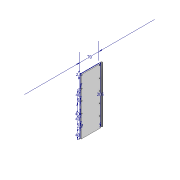
# Autodesk Inventor part: SidePanel
Saved by Autodesk Inventor 2020.3 (Build 243373010, 373A)
## iProperties
Created: 2020-12-03
Part Number: SidePanel
Material: Generic
Document SubType Name: Modeling
Designer: Yusuf
Mass: 79.5373 g
Surface Area: 369.992 cm^2
Volume: 79.5373 cm^3
Density: 1 g/cm^3
Appearance: Default
Author: Yusuf
Autodesk Inventor part; units mm, degrees
ref_plane "YZ Plane" through (0, 0, 0) normal (1, 0, 0) x (0, 1, 0)
ref_plane "XZ Plane" through (0, 0, 0) normal (0, 1, 0) x (-1, 0, 0)
ref_plane "XY Plane" through (0, 0, 0) normal (0, 0, 1) x (1, 0, 0)
sketch "Sketch1" plane through (0, 0, 0) normal (1, 0, 0) x (0, 1, 0)
  line L0 (0, 0) -> (205, 0)
  line L1 (205, 0) -> (205, -70)
  line L2 (205, -70) -> (0, -70)
  line L3 (0, -70) -> (0, 0)
  circle A0 centre (40, -2.5) radius 1
  circle A1 centre (80, -2.5) radius 1
  circle A2 centre (120, -2.5) radius 1
  circle A3 centre (160, -2.5) radius 1
  line L4 (0, 0) -> (0, 5)
  circle A4 centre (202.5, -2.5) radius 1.1944
  line L5 (0, -35) -> (205, -35) construction
  point P0 (40, -67.5)
  point P1 (80, -67.5)
  point P2 (120, -67.5)
  point P3 (160, -67.5)
  point P4 (202.5, -67.5)
  dimension "d0" = 205
  dimension "d1" = 70
  dimension "d2" = 2
  dimension "d3" = 2
  dimension "d4" = 2
  dimension "d5" = 2
  dimension "d7" = 40
  dimension "d8" = 40
  dimension "d9" = 40
  dimension "d10" = 2.5
  dimension "d11" = 40
  dimension "d12" = 2.5
  constraints: 12 end point, 5 centre point, 5 symmetric about line, 4 horizontal alignment, 2 midpoint, 2 parallel, 1 horizontal, 1 perpendicular
  measures "d0" distance of L1.end L2.end
  measures "d1" distance of L0.end L1.end
  measures "d2" diameter of A0
  measures "d3" diameter of A1
  measures "d4" diameter of A2
  measures "d5" diameter of A3
  measures "d7" distance of A3.centre A2.centre
  measures "d8" distance of A1.centre A2.centre
  measures "d9" distance of A1.centre A0.centre
  measures "d10" distance from line of L0 A0.centre
  measures "d11" distance from line of L3 A0.centre
  measures "d12" distance from line of L1 A4.centre
extrude "Extrusion1" add sketch "Sketch1" along normal blind 5 contours L0 L1 L2 L3 | A0 | A1 | A2 | A3 | A4
hole "Hole1" at (0, 202.5, -67.5) at (0, 160, -67.5) at (0, 120, -67.5) at (0, 80, -67.5) at (0, 40, -67.5) at (0, 40, -2.5) at (0, 80, -2.5) at (0, 120, -2.5) at (0, 160, -2.5) at (0, 202.5, -2.5) direction (1, 0, 0) diameter 3.242 depth 11.8 thread size "M4x0.7" class "6H" standard "ANSI Metric M Profile"
sketch "Sketch2" plane through (0, 0, -70) normal (0, 0, -1) x (-1, 0, 0)
  line L0 (0, 205) -> (0, 0) projected
  line L1 (-5, 205) -> (0, 205)
  line L2 (0, 205) -> (0, 0)
  line L3 (0, 0) -> (-5, 0)
  line L4 (-5, 0) -> (-5, 205)
  constraints: 8 end point, 2 parallel, 1 horizontal, 1 perpendicular
extrude "Extrusion2" add sketch "Sketch2" along normal blind 10
sketch "Sketch3" plane through (0, 0, 0) normal (0, -1, 0) x (1, 0, 0)
  line L0 (5, 0) -> (5, -80) projected
  line L1 (5, -80) -> (5, -70)
  line L2 (5, -77) -> (2.5, -77)
  line L3 (2.5, -77) -> (2.5, -73)
  line L4 (2.5, -73) -> (5, -73)
  line L5 (5, -80) -> (0, -80) projected
  point P0 (0, 0)
  dimension "d24" = 10
  dimension "d25" = 2.5
  dimension "d26" = 4
  dimension "d27" = 3
  constraints: 8 end point, 3 perpendicular, 3 point on line
  measures "d24" distance of L0.end L1.end
  measures "d25" distance of L2.start L2.end
  measures "d26" distance of L2.end L3.end
  measures "d27" distance between parallel lines of L5 L2
extrude "Extrusion3" cut sketch "Sketch3" against normal up to surface (205 mm away)
body "Solid1"
